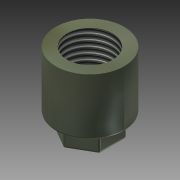
# Autodesk Inventor part: 水箱出水口盖
Saved by Autodesk Inventor 2015 (Build 190159000, 159)
## iProperties
Created: 2017-05-22
Part Number: 水箱出水口盖
Material: 常规
Document SubType Name: Modeling
Designer: Administrator
Density: 1 g/cm^3
Appearance: 预制平滑
Author: Administrator
Autodesk Inventor part; units mm, degrees
ref_plane "YZ Plane" through (0, 0, 0) normal (1, 0, 0) x (0, 1, 0)
ref_plane "XZ Plane" through (0, 0, 0) normal (0, 1, 0) x (-1, 0, 0)
ref_plane "XY Plane" through (0, 0, 0) normal (0, 0, 1) x (1, 0, 0)
sketch "草图1" plane through (0, 0, 0) normal (0, 0, 1) x (1, 0, 0)
  circle A0 centre (0, 0) radius 15
  dimension "d0" = 30
  constraints: 1 centre point, 1 coincident
  measures "d0" diameter of A0
extrude "拉伸1" add sketch "草图1" along normal blind 25
sketch "草图2" plane through (0, 0, 25) normal (0, 0, 1) x (1, 0, 0)
  circle A0 centre (0, 0) radius 10
  dimension "d3" = 20
  constraints: 1 centre point, 1 coincident
  measures "d3" diameter of A0
extrude "拉伸2" cut sketch "草图2" against normal blind 20
thread "螺纹1" size "M20x2.5" class "6H" standard "ANSI Metric M Profile" full length
sketch "草图3" plane through (0, 0, 0) normal (0, 0, -1) x (-1, 0, 0)
  line L0 (10, 5.7735) -> (10, -5.7735)
  line L1 (10, -5.7735) -> (0, -11.547)
  line L2 (0, -11.547) -> (-10, -5.7735)
  line L3 (-10, -5.7735) -> (-10, 5.7735)
  line L4 (-10, 5.7735) -> (0, 11.547)
  line L5 (0, 11.547) -> (10, 5.7735)
  line L6 (0, 0) -> (-10, 0)
  dimension "d8" = 20
  constraints: 14 end point, 1 coincident, 1 horizontal, 1 midpoint, 13 other
  measures "d8" distance between parallel lines of L0 L3
extrude "拉伸3" add sketch "草图3" along normal blind 8
fillet "圆角1" radius 1 13 edges at (-15, 0, 0) (5, 8.6603, -8) (-5, 8.6603, -8) (-10, 0, -8) (-5, -8.6603, -8) (5, -8.6603, -8) (10, 0, -8) (10, 5.7735, -4) (0, 11.547, -4) (-10, 5.7735, -4) (-10, -5.7735, -4) (0, -11.547, -4) (10, -5.7735, -4)
